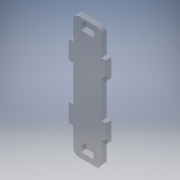
# Autodesk Inventor part: Back_Wall
Saved by Autodesk Inventor 2016 (Build 200138000, 138)
## iProperties
Created: 2015-06-25
Part Number: Back_Wall
Material: Generic
Document SubType Name: Modeling
Designer: Openlab
Density: 1 g/cm^3
Appearance: Polycarbonate - Clear
Author: Openlab
Autodesk Inventor part; units mm, degrees
ref_plane "YZ Plane" through (0, 0, 0) normal (1, 0, 0) x (0, 1, 0)
ref_plane "XZ Plane" through (0, 0, 0) normal (0, 1, 0) x (-1, 0, 0)
ref_plane "XY Plane" through (0, 0, 0) normal (0, 0, 1) x (1, 0, 0)
sketch "Sketch1" plane through (0, 0, 0) normal (0, 1, 0) x (-1, 0, 0)
  line L0 (7.75, -19.9274) -> (7.75, -42.3236) construction
  line L1 (13.2323, -33.5) -> (6.4845, -33.5) construction
  line L2 (15.5, -13.5) -> (17.95, -13.5)
  line L3 (17.95, -13.5) -> (17.95, -23.5)
  line L4 (17.95, -23.5) -> (15.5, -23.5)
  line L5 (15.5, -43.5) -> (17.95, -43.5)
  line L6 (17.95, -43.5) -> (17.95, -53.5)
  line L7 (17.95, -53.5) -> (15.5, -53.5)
  line L8 (0, -13.5) -> (-2.45, -13.5)
  line L9 (-2.45, -13.5) -> (-2.45, -23.5)
  line L10 (-2.45, -23.5) -> (0, -23.5)
  line L11 (0, -43.5) -> (-2.45, -43.5)
  line L12 (-2.45, -53.5) -> (0, -53.5)
  line L13 (-2.45, -53.5) -> (-2.45, -43.5)
  line L14 (15.5, -13.5) -> (15.5, -3)
  line L15 (15.5, -64) -> (15.5, -53.5)
  line L16 (15.5, -43.5) -> (15.5, -23.5)
  line L17 (0, -3) -> (0, -13.5)
  line L18 (0, -23.5) -> (0, -43.5)
  line L19 (0, -53.5) -> (0, -64)
  line L20 (12.5, 0) -> (3, 0)
  line L21 (3, -67) -> (12.5, -67)
  line L22 (11.25, -3) -> (4.25, -3)
  line L23 (4.25, -3) -> (4.25, -6)
  line L24 (4.25, -6) -> (11.25, -6)
  line L25 (11.25, -6) -> (11.25, -3)
  line L26 (11.25, -61) -> (4.25, -61)
  line L27 (4.25, -61) -> (4.25, -64)
  line L28 (4.25, -64) -> (11.25, -64)
  line L29 (11.25, -64) -> (11.25, -61)
  arc A0 (15.5, -3) -> (12.5, 0) centre (12.5, -3) ccw
  arc A1 (3, 0) -> (0, -3) centre (3, -3) ccw
  arc A2 (12.5, -67) -> (15.5, -64) centre (12.5, -64) ccw
  arc A3 (0, -64) -> (3, -67) centre (3, -64) ccw
  point P0 (0, 0)
  dimension "d8" = 10
  dimension "d9" = 20
  dimension "d17" = 2.45
  dimension "d21" = 67
  dimension "d22" = 15.5
  dimension "d23" = 7
  dimension "d24" = 3
  dimension "d25" = 3
  dimension "d27" = 6
  constraints: 60 end point, 15 parallel, 14 perpendicular, 12 point on line, 8 point on circle, 8 tangent, 6 horizontal, 5 collinear, 4 centre point, 3 equal length, 3 equal radius, 1 vertical, 6 other
  measures "d8" distance of L2.end L3.end
  measures "d9" distance between parallel lines of L5 L4
  measures "d17" distance of L8.start L8.end
  measures "d21" distance between parallel lines of L21 L20
  measures "d22" distance between parallel lines of L18 L16
  measures "d23" distance of L23.end L24.end
  measures "d24" distance of L24.end L22.start
  measures "d25" distance between parallel lines of L21 L28
  measures "d27" diameter of A1
extrude "Extrusion1" add sketch "Sketch1" along normal blind 3
body "Solid1"
